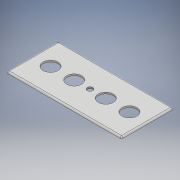
# Autodesk Inventor part: Cover
Saved by Autodesk Inventor 2018.3 (Build 223285000, 285)
## iProperties
Created: 2022-01-12
Part Number: Cover
Material: Generic
Document SubType Name: Modeling
Designer: Michael
Density: 1 g/cm^3
Appearance: Default
Author: Michael
Autodesk Inventor part; units mm, degrees
ref_plane "YZ Plane" through (0, 0, 0) normal (1, 0, 0) x (0, 1, 0)
ref_plane "XZ Plane" through (0, 0, 0) normal (0, 1, 0) x (-1, 0, 0)
ref_plane "XY Plane" through (0, 0, 0) normal (0, 0, 1) x (1, 0, 0)
sketch "Sketch1" plane through (0, 0, 0) normal (0, 0, 1) x (1, 0, 0)
  line L0 (-73, -33) -> (73, -33)
  line L1 (73, -33) -> (73, 33)
  line L2 (73, 33) -> (-73, 33)
  line L3 (-73, 33) -> (-73, -33)
  line L4 (-73, -33) -> (73, 33) construction
  line L5 (73, -33) -> (-73, 33) construction
  circle A0 centre (-20, 0) radius 9.5
  circle A1 centre (-50, 0) radius 9.5
  circle A2 centre (20, 0) radius 9.5
  circle A3 centre (50, 0) radius 9.5
  circle A4 centre (0, 0) radius 3.5
  dimension "d0" = 146
  dimension "d1" = 66
  dimension "d2" = 19
  dimension "d3" = 30
  dimension "d4" = 30
  dimension "d5" = 40
  dimension "d6" = 20
  dimension "d7" = 0
  dimension "d8" = 0
  dimension "d9" = 0
  dimension "d10" = 0
  dimension "d11" = 7
  constraints: 12 end point, 5 centre point, 3 equal radius, 2 midpoint, 2 parallel, 1 coincident, 1 horizontal, 1 perpendicular
  measures "d0" distance of L2.end L1.end
  measures "d1" distance of L1.end L0.end
  measures "d2" diameter of A1
  measures "d3" distance of A0.centre A1.centre
  measures "d4" distance of A2.centre A3.centre
  measures "d5" distance of A2.centre A0.centre
  measures "d6" distance of point (0, 0) A0.centre
  measures "d7" vertical distance of point (0, 0) A0.centre
  measures "d8" vertical distance of point (0, 0) A1.centre
  measures "d9" vertical distance of point (0, 0) A2.centre
  measures "d10" vertical distance of point (0, 0) A3.centre
  measures "d11" diameter of A4
extrude "Extrusion1" add sketch "Sketch1" along normal blind 2
fillet "Fillet1" radius 2 4 edges at (0, -33, 2) (73, 0, 2) (0, 33, 2) (-73, 0, 2)
fillet "Fillet2" radius 2 4 edges at (-72.4142, -32.4142, 1.4142) (-72.4142, 32.4142, 1.4142) (72.4142, 32.4142, 1.4142) (72.4142, -32.4142, 1.4142)
equation "\"d4\" = d3"
body "Solid1"
